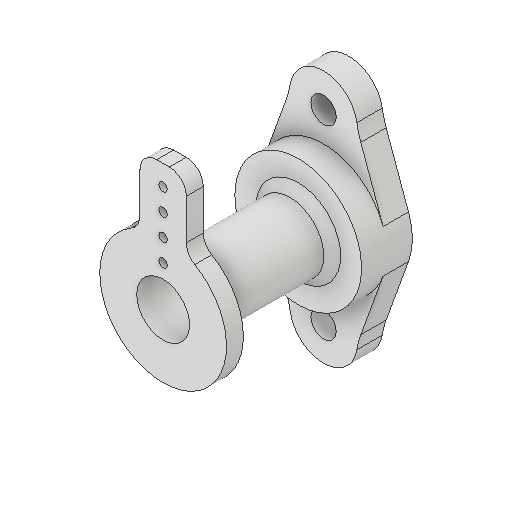
# Autodesk Inventor part: 3DP_ABS_Solenoid_Actuator_Body
Saved by Autodesk Inventor 2026.1 (Build 301233000, 233)
## iProperties
Created: 2018-06-14
Part Number: 3DP_ABS_Solenoid_Actuator_Body
Material: ABS Plastic
Document SubType Name: Modeling
Designer: Andrzej
Density: 1.06 g/cm^3
Appearance: Smooth - White
Author: Andrzej
Autodesk Inventor part; units mm, degrees
note: some values were not read from the file. Chosen so that the rebuilt part matches the saved one: sketch regions of "Extrusion4".
ref_plane "YZ Plane" through (0, 0, 0) normal (1, 0, 0) x (0, 1, 0)
ref_plane "XZ Plane" through (0, 0, 0) normal (0, 1, 0) x (-1, 0, 0)
ref_plane "XY Plane" through (0, 0, 0) normal (0, 0, 1) x (1, 0, 0)
sketch "Sketch1" plane through (0, 0, 0) normal (0, 0, 1) x (1, 0, 0)
  circle A0 centre (0, 0) radius 3.125
  circle A1 centre (0, 0) radius 4.025
  circle A2 centre (0, 0) radius 7.5
  dimension "d0" = 6.25
  dimension "d1" = 0.9
  dimension "d2" = 15
  constraints: 3 centre point, 2 coincident
  measures "d0" diameter of A0
  measures "d1" radial gap between concentric circles of A0 A1
  measures "d2" diameter of A2
extrude "Extrusion1" add sketch "Sketch1" along normal blind 2 contours A1 | A2
extrude "Extrusion2" add sketch "Sketch1" against normal blind 16 contours A1
sketch "Sketch2" plane through (0, 0, -16) normal (0, 0, -1) x (-1, 0, 0)
  circle A0 centre (0, 0) radius 4.025 projected
  circle A1 centre (0, 0) radius 7.5 projected
  circle A2 centre (0, 0) radius 3.125 projected
  circle A3 centre (0, 0) radius 1.5
  dimension "d9" = 3
  constraints: 1 centre point, 1 coincident
  measures "d9" diameter of A3
extrude "Extrusion3" add sketch "Sketch2" along normal blind 4 contours A0 | A1 | A2
sketch "Sketch3" plane through (0, 0, -20) normal (0, 0, -1) x (-1, 0, 0)
  circle A0 centre (0, 0) radius 1.5 projected
  circle A1 centre (0, 0) radius 7.5 projected
  circle A2 centre (0, 11) radius 1.5
  circle A3 centre (0, 11) radius 4
  circle A4 centre (0, 0) radius 7.5 projected
  line L0 (4, 11) -> (7.0537, 2.5487)
  line L1 (-4, 11) -> (-7.0537, 2.5487)
  dimension "d10" = 3
  dimension "d11" = 11
  dimension "d12" = 8
  dimension "d41" = 0
  constraints: 4 end point, 4 point on circle, 2 centre point, 2 tangent, 1 coincident
  measures "d10" diameter of A2
  measures "d11" distance of A2.centre point (0, 0)
  measures "d12" diameter of A3
  measures "d41" horizontal distance of point (0, 0) A2.centre
extrude "Extrusion4" add sketch "Sketch3" against normal blind 3
pattern_circular "Circular Pattern1" count 2 over 360 about axis through (0, 0, -16) along (0, 0, -1) of "Extrusion4"
extrude "Extrusion5" add sketch "Sketch2" against normal blind 2 contours A1
fillet "Fillet1" radius 10 4 edges at (-4, 11, -18.5) (4, 11, -18.5) (-4, -11, -18.5) (4, -11, -18.5)
chamfer "Chamfer1" distance 1 angle 45 2 edges at (-4.025, 0, -14) (-4.025, 0, 0)
sketch "Sketch4" plane through (0, 0, 2) normal (0, 0, 1) x (1, 0, 0)
  circle A0 centre (0, 0) radius 3.125 projected
  circle A1 centre (0, 0) radius 7.5 projected
  circle A2 centre (0, 0) radius 7.5 projected
  line L0 (2.75, 6.9776) -> (2.75, 15)
  line L1 (2.75, 15) -> (-2.75, 15)
  line L2 (-2.75, 15) -> (-2.75, 6.9776)
  circle A3 centre (0, 4.8) radius 0.5
  circle A4 centre (0, 7.4) radius 0.5
  circle A5 centre (0, 10) radius 0.5
  circle A6 centre (0, 12.6) radius 0.5
  circle A7 centre (0, 0) radius 4.025 projected
  dimension "d24" = 2.75
  dimension "d25" = 2.75
  dimension "d26" = 7.5
  dimension "d27" = 1
  dimension "d28" = 4.8
  dimension "d31" = 2.6
  constraints: 6 end point, 4 centre point, 2 perpendicular, 2 point on circle, 2 vertical, 6 other
  measures "d24" distance from line of point (0, 0) L0
  measures "d25" distance from line of point (0, 0) L2
  measures "d26" distance edge to line of A1 L1
  measures "d27" diameter of A3
  measures "d28" distance of point (0, 0) A3.centre
  measures "d31" distance of A3.centre A4.centre
extrude "Extrusion6" add sketch "Sketch4" against normal blind 2 contours A1 A4 L2 L1 L0 | A1 A4 picked at (0, 7.6321)
extrude "Extrusion7" cut sketch "Sketch4" against normal blind 3 contours A4 A1 | A1 A4 | A3 picked at (-0.014, 7.2994) picked at (0, 7.6321)
fillet "Fillet2" radius 2 4 edges at (2.75, 6.9776, 1) (-2.75, 6.9776, 1) (-2.75, 15, 1) (2.75, 15, 1)
equation "\"d25\" = d24"
body "Solid1"
